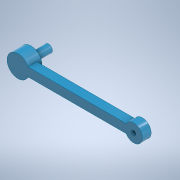
# Autodesk Inventor part: Rod
Saved by Autodesk Inventor 2020 (Build 240168000, 168)
## iProperties
Created: 2021-12-26
Part Number: Rod
Material: ABS Plastic
Document SubType Name: Modeling
Designer: Umur Batuhan Özmen
Density: 1.06 g/cm^3
Appearance: Sky Blue Dark
Author: Umur Batuhan Özmen
Autodesk Inventor part; units mm, degrees
ref_plane "YZ Plane" through (0, 0, 0) normal (1, 0, 0) x (0, 1, 0)
ref_plane "XZ Plane" through (0, 0, 0) normal (0, 1, 0) x (-1, 0, 0)
ref_plane "XY Plane" through (0, 0, 0) normal (0, 0, 1) x (1, 0, 0)
sketch "Sketch1" plane through (0, 0, 0) normal (0, 0, 1) x (1, 0, 0)
  circle A0 centre (0, 0) radius 12.5
  circle A1 centre (0, 0) radius 4.5
  arc A2 (123.8397, -5) -> (123.8397, 5) centre (132.5, 0) ccw
  line L0 (11.4564, 5) -> (123.8397, 5)
  line L1 (12.5, -5) -> (123.8397, -5)
  line L2 (12.5, -5) -> (11.4564, -5)
  circle A3 centre (132.5, 0) radius 2.5
  dimension "d0" = 25
  dimension "d1" = 9
  dimension "d3" = 20
  dimension "d6" = 5
  constraints: 6 end point, 4 centre point, 4 point on circle, 3 coincident, 1 parallel, 1 point on line
  measures "d0" diameter of A0
  measures "d1" diameter of A1
  measures "d3" diameter of A2
  measures "d6" diameter of A3
extrude "Extrusion1" add sketch "Sketch1" along normal blind 10 contours A0 | A0 L0 A2 L1 L2 | A1
extrude "Extrusion2" add sketch "Sketch1" against normal blind 5 contours A0
extrude "Extrusion3" add sketch "Sketch1" against normal blind 25 contours A1
body "Solid1"
